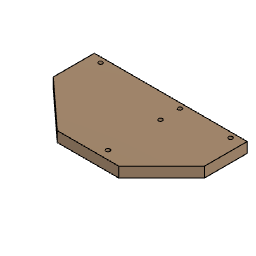
Brace TL (Autodesk Fusion 360 design; units mm, degrees)
Autodesk Fusion 360 part; units mm, degrees
sketch "Top" plane through (0, 0, 0) normal (0, 0, 1) x (1, 0, 0)
  line L0 (109, 75) -> (-159, 75)
  line L1 (-159, 75) -> (-159, 3)
  line L2 (-74, -75) -> (34, -75)
  line L3 (109, 0) -> (109, 75)
  line L4 (109, 0) -> (34, -75)
  line L5 (-159, 3) -> (-74, -75)
  line L6 (-159, 66) -> (109, 66) construction
  line L7 (0, 75) -> (0, -75) construction
  circle A0 centre (0, 66) radius 3.5
  circle A1 centre (0, 32) radius 3.5
  circle A2 centre (0, -60) radius 3.5
  circle A3 centre (89, 66) radius 3.5
  circle A4 centre (-139, 66) radius 3.5
  dimension "d3" = 75
  dimension "d5" = 75
  dimension "d6" = 85
  dimension "d7" = 78
  dimension "d9" = 159
  dimension "d11" = 268
  dimension "d12" = 9
  dimension "d13" = 109
  dimension "d14" = 7
  dimension "d15" = 7
  dimension "d16" = 7
  dimension "d17" = 34
  dimension "d18" = 92
  dimension "d19" = 7
  dimension "d20" = 7
  dimension "d21" = 89
  dimension "d22" = 139
  dimension "d23" = 150
  constraint perpendicular L0 L1
  constraint parallel L0 L2
  constraint parallel L1 L3
  constraint horizontal L0
  constraint coincident L1 L6.start
  constraint coincident L3 L6.end
  constraint perpendicular L3 L6
  constraint coincident L0 L7.start
  constraint coincident L2 L7.end
  constraint perpendicular L2 L7
  constraint coincident L7 A0.centre
  constraint coincident L6 A0.centre
  constraint coincident L7 A1.centre
  constraint coincident L7 A2.centre
  constraint coincident L6 A3.centre
  constraint coincident L6 A4.centre
  measures "d3" horizontal distance of L3.start L2.end
  measures "d5" vertical distance of L3.start L2.end
  measures "d6" horizontal distance of L1.end L2.start
  measures "d7" vertical distance of L1.end L2.start
  measures "d9" distance of origin L1
  measures "d11" distance of L0.start L0.end
  measures "d12" distance of L0 L6
  measures "d13" distance of L3 L7
  measures "d14" diameter of A0
  measures "d15" diameter of A1
  measures "d16" diameter of A2
  measures "d17" distance of A0.centre A1.centre
  measures "d18" distance of A1.centre A2.centre
  measures "d19" diameter of A3
  measures "d20" diameter of A4
  measures "d21" distance of A0.centre A3.centre
  measures "d22" distance of A0.centre A4.centre
  measures "d23" distance of L0 L2
extrude "Extrude1" add sketch "Top" along normal blind 18
named bodies: "Brace TL"
